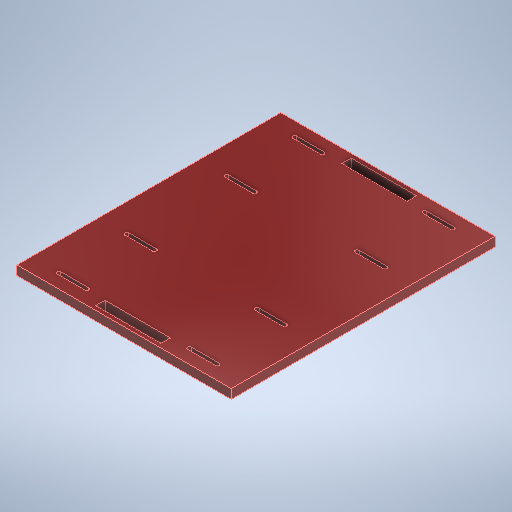
# Autodesk Inventor part: floor
Saved by Autodesk Inventor 2025.3 (Build 293356030, 356C)
## iProperties
Created: 2026-06-25
Part Number: floor
Material: Brass, Soft Yellow
Document SubType Name: Modeling
Designer: user
Density: 8.47 g/cm^3
Appearance: High Gloss - Burnt Red
Author: user
Autodesk Inventor part; units mm, degrees
ref_plane "YZ Plane" through (0, 0, 0) normal (1, 0, 0) x (0, 1, 0)
ref_plane "XZ Plane" through (0, 0, 0) normal (0, 1, 0) x (-1, 0, 0)
ref_plane "XY Plane" through (0, 0, 0) normal (0, 0, 1) x (1, 0, 0)
sketch "Sketch1" plane through (0, 0, 0) normal (0, 1, 0) x (-1, 0, 0)
  line L0 (-229.8634, 7.9265) -> (-229.8634, -272.0735)
  line L1 (0, -264.1469) -> (0, 0)
  line L2 (-114.9317, 7.8456) -> (-114.9317, -271.9925) construction
  line L3 (-229.8634, -132.0735) -> (0, -132.0735) construction
  line L4 (0, -222.0735) -> (-229.8634, -222.0735) construction
  line L5 (0.0192, -20.1711) -> (0, -20.138) construction
  line L6 (0.9366, -42.0735) -> (-229.8634, -42.0735) construction
  line L7 (-39.8418, -42.0735) -> (-39.8418, -2.1597) construction
  line L8 (-39.8418, -5.776) -> (-30, -5.776)
  line L9 (-39.8418, -5.776) -> (-60, -5.776)
  line L10 (-30, -5.776) -> (-60, -5.776) construction
  line L11 (-30, -3.776) -> (-60, -3.776)
  line L12 (-60, -7.776) -> (-30, -7.776)
  arc A0 (-30, -7.776) -> (-30, -3.776) centre (-30, -5.776) ccw
  arc A1 (-60, -3.776) -> (-60, -7.776) centre (-60, -5.776) ccw
  line L13 (-39.8418, -78.371) -> (-30, -78.371)
  line L14 (-39.8418, -78.371) -> (-60, -78.371)
  line L15 (-30, -78.371) -> (-60, -78.371) construction
  line L16 (-30, -80.371) -> (-60, -80.371)
  line L17 (-60, -76.371) -> (-30, -76.371)
  arc A2 (-30, -80.371) -> (-30, -76.371) centre (-30, -78.371) ccw
  arc A3 (-60, -76.371) -> (-60, -80.371) centre (-60, -78.371) ccw
  line L18 (-231.5784, -23.0949) -> (-148.4647, -23.0949) construction
  line L19 (-148.4647, -23.0949) -> (-148.4647, -61.0949) construction
  line L20 (-148.4647, -61.0949) -> (-231.5784, -61.0949) construction
  line L21 (-190.0216, -5.776) -> (-199.8634, -5.776)
  line L22 (-190.0216, -5.776) -> (-169.8634, -5.776)
  line L23 (-199.8634, -5.776) -> (-169.8634, -5.776) construction
  line L24 (-199.8634, -3.776) -> (-169.8634, -3.776)
  line L25 (-169.8634, -7.776) -> (-199.8634, -7.776)
  arc A4 (-199.8634, -3.776) -> (-199.8634, -7.776) centre (-199.8634, -5.776) ccw
  arc A5 (-169.8634, -7.776) -> (-169.8634, -3.776) centre (-169.8634, -5.776) ccw
  arc A6 (-169.8634, -80.371) -> (-169.8634, -76.371) centre (-169.8634, -78.371) ccw
  line L26 (-190.0216, -78.371) -> (-169.8634, -78.371)
  line L27 (-169.8634, -76.371) -> (-199.8634, -76.371)
  line L28 (-190.0216, -78.371) -> (-199.8634, -78.371)
  line L29 (-199.8634, -78.371) -> (-169.8634, -78.371) construction
  line L30 (-199.8634, -80.371) -> (-169.8634, -80.371)
  arc A7 (-199.8634, -76.371) -> (-199.8634, -80.371) centre (-199.8634, -78.371) ccw
  line L31 (-114.9317, -271.9925) -> (-114.9317, 7.8456) construction
  line L32 (0, -222.0735) -> (-229.8634, -222.0735) construction
  line L33 (-15.354, -241.052) -> (-98.4678, -241.052) construction
  line L34 (-98.4678, -241.052) -> (-98.4678, -203.052) construction
  line L35 (-98.4678, -203.052) -> (-15.354, -203.052) construction
  line L36 (-39.8418, -222.0735) -> (-39.8418, -261.9872) construction
  line L37 (-39.8418, -258.371) -> (-30, -258.371)
  line L38 (-39.8418, -258.371) -> (-60, -258.371)
  line L39 (-30, -258.371) -> (-60, -258.371) construction
  line L40 (-30, -260.371) -> (-60, -260.371)
  line L41 (-60, -256.371) -> (-30, -256.371)
  arc A8 (-30, -260.371) -> (-30, -256.371) centre (-30, -258.371) ccw
  arc A9 (-60, -256.371) -> (-60, -260.371) centre (-60, -258.371) ccw
  arc A10 (-60, -183.776) -> (-60, -187.776) centre (-60, -185.776) ccw
  line L42 (-39.8418, -185.776) -> (-60, -185.776)
  line L43 (-60, -187.776) -> (-30, -187.776)
  line L44 (-39.8418, -185.776) -> (-30, -185.776)
  line L45 (-30, -185.776) -> (-60, -185.776) construction
  line L46 (-30, -183.776) -> (-60, -183.776)
  arc A11 (-30, -187.776) -> (-30, -183.776) centre (-30, -185.776) ccw
  line L47 (-148.4647, -241.052) -> (-148.4647, -203.052) construction
  line L48 (-169.8634, -256.371) -> (-199.8634, -256.371)
  line L49 (-190.0216, -258.371) -> (-199.8634, -258.371)
  line L50 (-190.0216, -258.371) -> (-169.8634, -258.371)
  arc A12 (-199.8634, -256.371) -> (-199.8634, -260.371) centre (-199.8634, -258.371) ccw
  line L51 (-199.8634, -260.371) -> (-169.8634, -260.371)
  arc A13 (-169.8634, -260.371) -> (-169.8634, -256.371) centre (-169.8634, -258.371) ccw
  line L52 (-199.8634, -258.371) -> (-169.8634, -258.371) construction
  line L53 (-169.8634, -187.776) -> (-199.8634, -187.776)
  line L54 (-190.0216, -185.776) -> (-199.8634, -185.776)
  arc A14 (-199.8634, -183.776) -> (-199.8634, -187.776) centre (-199.8634, -185.776) ccw
  line L55 (-199.8634, -185.776) -> (-169.8634, -185.776) construction
  line L56 (-199.8634, -183.776) -> (-169.8634, -183.776)
  line L57 (-190.0216, -185.776) -> (-169.8634, -185.776)
  arc A15 (-169.8634, -187.776) -> (-169.8634, -183.776) centre (-169.8634, -185.776) ccw
  line L58 (-148.4647, -203.052) -> (-231.5784, -203.052) construction
  line L59 (-231.5784, -241.052) -> (-148.4647, -241.052) construction
  line L60 (-192.7799, 9.4375) -> (-30.2751, 9.4375)
  line L61 (-192.7799, -273.5844) -> (-30.2751, -273.5844)
  line L62 (-80, -5) -> (-150, -5)
  line L63 (-150, -5) -> (-150, 5)
  line L64 (-150, 5) -> (-80, 5)
  line L65 (-80, 5) -> (-80, -5)
  line L66 (-80, -259.1469) -> (-150, -259.1469)
  line L67 (-150, -259.1469) -> (-150, -269.1469)
  line L68 (-150, -269.1469) -> (-80, -269.1469)
  line L69 (-80, -269.1469) -> (-80, -259.1469)
  line L70 (0, 0) -> (0, 9.4375)
  line L71 (0, 9.4375) -> (-30.2751, 9.4375)
  line L72 (-192.7799, 9.4375) -> (-229.8634, 9.4375)
  line L73 (-229.8634, 9.4375) -> (-229.8634, 7.9265)
  line L74 (0, -264.1469) -> (0, -273.5844)
  line L75 (0, -273.5844) -> (-30.2751, -273.5844)
  line L76 (-192.7799, -273.5844) -> (-229.8634, -273.5844)
  line L77 (-229.8634, -273.5844) -> (-229.8634, -272.0735)
  point P0 (-39.8418, -23.0949)
  point P1 (-45, -5.776)
  point P2 (-45, -78.371)
  point P3 (-190.0216, -42.0735)
  point P4 (-190.0216, -23.0949)
  point P5 (-184.8634, -5.776)
  point P6 (-184.8634, -78.371)
  point P7 (-39.8418, -241.052)
  point P8 (-45, -258.371)
  point P9 (-45, -185.776)
  point P10 (-190.0216, -222.0735)
  point P11 (-190.0216, -241.052)
  point P12 (-184.8634, -185.776)
  point P13 (-184.8634, -258.371)
  point P14 (-114.9317, 2.9056)
  point P15 (-45, -78.371)
  point P16 (-45, -185.776)
  point P17 (-114.9317, -267.0525)
  point P18 (-184.8634, -185.776)
  point P19 (-45, -258.371)
  point P20 (-229.8634, -272.8289)
  dimension "d25" = 4
  dimension "d34" = 30
  dimension "d36" = 280
  dimension "d47" = 45
  dimension "d49" = 45
  dimension "d50" = 45
  dimension "d51" = 229.8634
  constraints: 172 end point, 78 symmetric about line, 32 point on circle, 16 centre point, 11 point on line, 8 midpoint, 5 perpendicular, 4 parallel, 4 tangent, 3 collinear, 3 horizontal, 2 vertical, 14 other
  measures "d25" distance of L12.end L11.start
  measures "d34" distance of L9.end L8.end
  measures "d36" distance of L0.start L0.end
  measures "d47" distance from line of L0 point (-184.863, -185.776)
  measures "d49" distance from line of L1 point (-45, -258.371)
  measures "d50" distance from line of L1 point (-45, -185.776)
  measures "d51" horizontal distance of point (-229.863, -272.829) L74.end
extrude "Extrusion1" add sketch "Sketch1" along normal blind 10 contours L73 L72 L60 L71 L70 L1 L74 L75 L61 L76 L77 L0 | A0 L12 A1 L11 | L16 A3 L17 A2 | L24 A5 L25 A4 | L30 A7 L27 A6 | L40 A9 L41 A8 | L46 A11 L43 A10 | A13 L51 A12 L48 | L53 A14 L56 A15 | L62 L63 L64 L65 | L69 L68 L67 L66
extrude "Extrusion2" cut sketch "Sketch1" along normal through all contours A0 L12 A1 L11 | L16 A3 L17 A2 | L24 A5 L25 A4 | L30 A7 L27 A6 | L40 A9 L41 A8 | L46 A11 L43 A10 | A13 L51 A12 L48 | L53 A14 L56 A15
extrude "Extrusion4" add sketch "Sketch1" along normal blind 10 contours L73 L72 L60 L71 L70 L1 L74 L75 L61 L76 L77 L0 | A0 L12 A1 L11 | L16 A3 L17 A2 | L24 A5 L25 A4 | L30 A7 L27 A6 | L40 A9 L41 A8 | L46 A11 L43 A10 | A13 L51 A12 L48 | L53 A14 L56 A15 | L62 L63 L64 L65 | L69 L68 L67 L66
extrude "Extrusion5" cut sketch "Sketch1" along normal blind 10 contours L62 L63 L64 L65 | L69 L68 L67 L66
extrude "Extrusion6" cut sketch "Sketch1" along normal blind 10 contours L24 A5 L25 A4
extrude "Extrusion7" cut sketch "Sketch1" along normal blind 10 contours A0 L12 A1 L11 | L16 A3 L17 A2 | L30 A7 L27 A6 | L40 A9 L41 A8 | L46 A11 L43 A10 | A13 L51 A12 L48 | L53 A14 L56 A15
body "Solid1"
